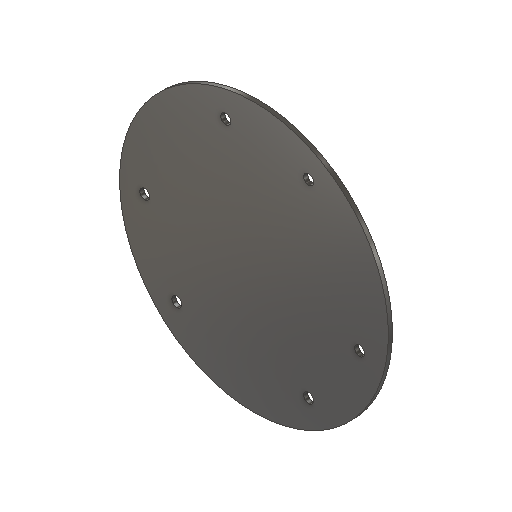
# Autodesk Inventor part: CNCM_STEEL_Bowl_Electromagnet_Plate
Saved by Autodesk Inventor 2026.1 (Build 301233000, 233)
## iProperties
Created: 2018-05-27
Part Number: CNCM_STEEL_Bowl_Electromagnet_Plate
Material: Steel
Document SubType Name: Modeling
Designer: Andrzej
Density: 7.85 g/cm^3
Appearance: Steel - Polished
Author: Andrzej
Autodesk Inventor part; units mm, degrees
ref_plane "YZ Plane" through (0, 0, 0) normal (1, 0, 0) x (0, 1, 0)
ref_plane "XZ Plane" through (0, 0, 0) normal (0, 1, 0) x (-1, 0, 0)
ref_plane "XY Plane" through (0, 0, 0) normal (0, 0, 1) x (1, 0, 0)
sketch "Sketch1" plane through (0, 0, 0) normal (0, 0, 1) x (1, 0, 0)
  circle A0 centre (0, 0) radius 40
  circle A1 centre (0, 0) radius 32.5
  line L0 (0, 0) -> (-26.7142, -26.7142)
  line L1 (0, 0) -> (37.7796, 0) construction
  point P0 (-32.5, 0)
  point P1 (-32.5, 0)
  point P2 (-22.981, -22.981)
  point P3 (-32.5, 0)
  dimension "d0" = 80
  dimension "d1" = 65
  dimension "d3" = 135
  constraints: 4 coincident, 4 end point, 2 centre point, 2 point on circle, 1 equal length, 1 horizontal, 1 point on line
  measures "d0" diameter of A0
  measures "d1" diameter of A1
  measures "d3" angle of L0 L1
extrude "Extrusion1" add sketch "Sketch1" along normal blind 1.2 contours A0 | A1
hole "Hole1" at (-32.5, 0, 0) at (-22.981, -22.981, 0) direction (0, 0, 1) diameter 3 end through all
pattern_circular "Circular Pattern1" count 3 over 360 about axis through (0, 0, -10) along (0, 0, 1) of "Hole1"
body "Solid1"
